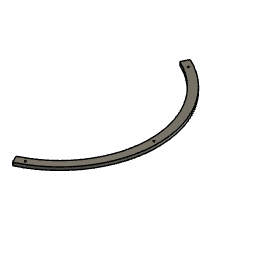
move_base_bumper_front (Autodesk Fusion 360 design; units mm, degrees)
Autodesk Fusion 360 part; units mm, degrees
note: some values were not read from the file. Set by a fixed rule: the direction of a hole.
sketch "スケッチ1" plane through (0, 0, 0) normal (0, 1, 0) x (1, 0, 0)
  arc A0 (77.7618, -166.7606) -> (77.7618, 166.7606) centre (0, 0) ccw
  arc A1 (84.5237, -181.2616) -> (84.5237, 181.2616) centre (0, 0) ccw
  line L0 (84.5237, 181.2616) -> (0, 0)
  line L1 (0, 0) -> (84.5237, -181.2616)
  arc A2 (96, -166.2769) -> (96, 166.2769) centre (0, 0) ccw
  line L2 (96, 166.2769) -> (0, 0)
  line L3 (96, -166.2769) -> (0, 0)
  line L4 (0, 0) -> (192, 0)
  dimension "d1" = 200
  dimension "d2" = 184
  dimension "d3" = 192
  dimension "d4" = 60
  dimension "d5" = 60
  dimension "d6" = 65
  dimension "d8" = 65
  constraint coincident A0.centre A1.centre
  constraint coincident A0.end L0
  constraint coincident A0.start L1
  constraint coincident A2 L4.end
  constraint horizontal L4
  measures "d1" radius of A1
  measures "d2" radius of A0
  measures "d3" radius of A2
  measures "d4" angle of L2 L4
  measures "d5" angle of L3 L4
  measures "d6" angle of L1 L4
  measures "d8" angle of L0 L4
extrude "押し出し1" add sketch "スケッチ1" along normal blind 6 contours A0 A1 L0 L1 A2 L2 L3 | A0 A2 L3 L4 | A0 A2 L2 L4
hole "穴1" at (192, 0, 0) at (96, 0, 166.2769) at (96, 0, -166.2769) direction (0, 1, 0) diameter 3.2 end through all
fillet "フィレット1" radius 1 4 edges at (84.5237, 3, 181.2616) (77.7618, 3, 166.7606) (84.5237, 3, -181.2616) (77.7618, 3, -166.7606)
